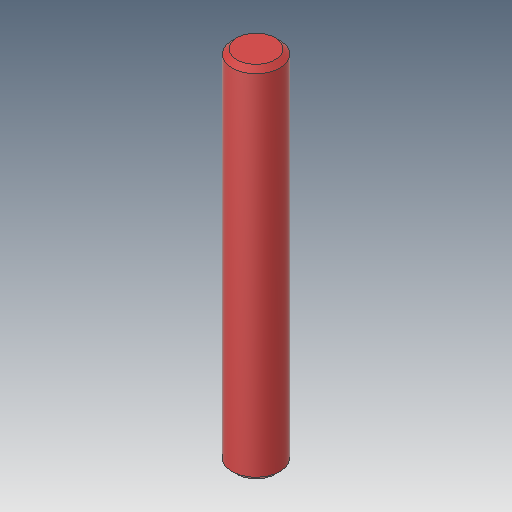
# Autodesk Inventor part: pin_2x15
Saved by Autodesk Inventor 2019.4 (Build 234330000, 330)
## iProperties
Created: 2018-07-27
Part Number: pin_2x15
Material: 鋼
Document SubType Name: Modeling
Designer: student
Density: 7.85 g/cm^3
Appearance: 滑らか - 赤
Mass: 0.368081 g
Surface Area: 0.989546 cm^2
Volume: 0.0468893 cm^3
Author: student
Autodesk Inventor part; units mm, degrees
ref_plane "YZ Plane" through (0, 0, 0) normal (1, 0, 0) x (0, 1, 0)
ref_plane "XZ Plane" through (0, 0, 0) normal (0, 1, 0) x (-1, 0, 0)
ref_plane "XY Plane" through (0, 0, 0) normal (0, 0, 1) x (1, 0, 0)
sketch "スケッチ1" plane through (0, 0, 0) normal (0, 1, 0) x (-1, 0, 0)
  circle A0 centre (0, 0) radius 1
  dimension "d0" = 2
  constraints: 1 centre point, 1 coincident
  measures "d0" diameter of A0
extrude "押し出し1" add sketch "スケッチ1" along normal mid plane 15
chamfer "面取り1" distance 0.2 angle 45 2 edges at (1, 7.5, 0) (1, -7.5, 0)
